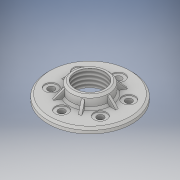
# Autodesk Inventor part: 2 Inch Pipe Flange
Saved by Autodesk Inventor 2019 (Build 230136000, 136)
## iProperties
Created: 2019-08-29
Part Number: 2 Inch Pipe Flange
Material: Generic
Document SubType Name: Modeling
Designer: Rick Szalay
Density: 1 g/cm^3
Appearance: Default
Author: Rick Szalay
Autodesk Inventor part; units mm, degrees
ref_plane "YZ Plane" through (0, 0, 0) normal (1, 0, 0) x (0, 1, 0)
ref_plane "XZ Plane" through (0, 0, 0) normal (0, 1, 0) x (-1, 0, 0)
ref_plane "XY Plane" through (0, 0, 0) normal (0, 0, 1) x (1, 0, 0)
sketch "Sketch1" plane through (0, 0, 0) normal (0, 0, 1) x (1, 0, 0)
  line L0 (0, 0) -> (0, 25.4)
  line L1 (0, 25.4) -> (-28.575, 25.4)
  line L2 (-28.575, 7.9375) -> (-63.5, 7.9375)
  line L3 (-63.5, 7.9375) -> (-63.5, 0)
  line L4 (-63.5, 0) -> (0, 0)
  line L5 (-28.575, 25.4) -> (-28.575, 7.9375)
  dimension "d1" = 7.9375
  dimension "d2" = 25.4
  dimension "d5" = 57.15
  dimension "d6" = 127
  constraints: 12 end point, 3 perpendicular, 2 vertical, 1 parallel
  measures "d1" distance between parallel lines of L2 L4
  measures "d2" distance between parallel lines of L4 L1
  measures "d5" diameter of L1.end L0
  measures "d6" diameter of L3 L0
revolve "Revolution1" add sketch "Sketch1" angle 360 about axis through (0, 0, 0) along (0, 1, 0)
sketch "Sketch2" plane through (0, 25.4, 0) normal (0, 1, 0) x (1, 0, 0)
  circle A0 centre (0, 0) radius 28.575 projected
  constraints: 1 coincident
hole "Hole1" at (0, 25.4, 0) direction (0, -1, 0) diameter 44.6786 end through all thread size "2-4.5 UNC" class "2B" standard "ANSI Unified Screw Threads"
sketch "Sketch3" plane through (0, 7.9375, 0) normal (0, 1, 0) x (1, 0, 0)
  circle A0 centre (0, 0) radius 63.5 construction
  circle A1 centre (0, 0) radius 22.3393 construction
  line L0 (0, 22.3393) -> (0, 42.9196) construction
  line L1 (0, 42.9196) -> (0, 63.5) construction
  circle A2 centre (0, 0) radius 63.5 construction
  line L2 (0, 63.5) -> (0, 0) construction
  dimension "d27" = 0
  constraints: 6 end point, 2 collinear, 2 point on circle, 1 point on line, 1 vertical, 1 vertical alignment, 1 other
  measures "d27" distance between parallel lines of L2 L1
hole "Hole2" at (0, 7.9375, -42.9196) direction (0, -1, 0) diameter 10.0838 end through all counterbore diameter 19.3548 counterbore depth 1.5875 clearance for "Flat Head Machine Screw (82)" size "3/8" standard "Ansi Unified Screw Threads"
sketch "Sketch5" plane through (0, 0, 0) normal (0, 0, 1) x (1, 0, 0)
  line L0 (-28.575, 7.9375) -> (-28.575, 25.4) projected
  line L1 (-28.575, 20.32) -> (-40.9575, 7.9375)
  line L2 (63.5, 7.9375) -> (-63.5, 7.9375) projected
  line L3 (28.575, 25.4) -> (-28.575, 25.4) projected
  point P0 (0, 0)
  dimension "d28" = 5.08
  dimension "d29" = 45
  constraints: 2 end point, 2 point on line
  measures "d28" distance from line of L1.start L3
  measures "d29" angle of L0 L1
extrude "Rib1" add sketch "Sketch5" along normal mid plane 3.81 rib yes fills toward (-34.7309, 14.0934) open curves L1
chamfer "Chamfer1" distance 3.175 angle 45 3 edges at (28.575, 25.4, 0) (63.5, 7.9375, 0) (28.575, 7.9375, 0)
pattern_circular "Circular Pattern2" count 6 over 360 about axis through (0, -155.9923, 0) along (0, 1, 0) of "Rib1", "Hole2"
body "Solid1"
